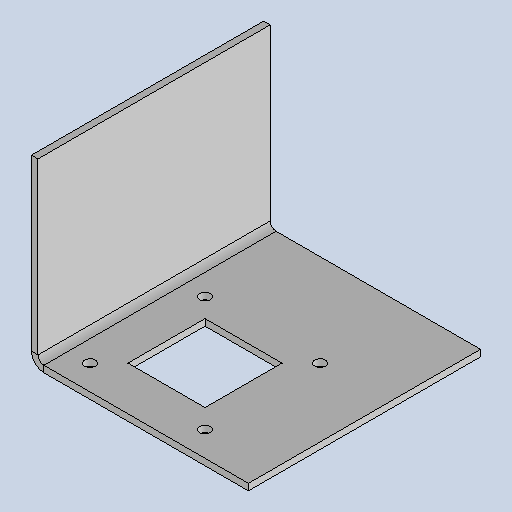
# Autodesk Inventor part: PNS 753 FDS 1200 FLANGE 2 up
Saved by Autodesk Inventor 2025.3 (Build 293356030, 356C)
## iProperties
Created: 2025-06-24
Part Number: PNS 753 FDS 1200 FLANGE 2 up
Material: Stainless Steel
Description: DIE16(5)|\ 90°|corrY -___°|X_____|bom___
Document SubType Name: Sheet Metal
Designer: pokla
Mass: 427.993 g
Surface Area: 379.976 cm^2
Volume: 53.4991 cm^3
Density: 8 g/cm^3
Flat Pattern Width: 17.8893 cm
Flat Pattern Length: 10.7 cm
Flat Pattern Area: 191.416 cm^2
Sheet Metal Rule: AISI304 2mm Die16
Sheet Metal Width: 178,893 mm
Sheet Metal Length: 107,000 mm
Sheet Metal Area: 19141,566 mm^2
Appearance: Default
d177: 30,000 mm
d178: 30,000 mm
Author: user
Autodesk Inventor part; units mm, degrees
ref_plane "YZ Plane" through (0, 0, 0) normal (1, 0, 0) x (0, 1, 0)
ref_plane "XZ Plane" through (0, 0, 0) normal (0, 1, 0) x (-1, 0, 0)
ref_plane "XY Plane" through (0, 0, 0) normal (0, 0, 1) x (1, 0, 0)
sketch "Sketch1" plane through (0, 0, 0) normal (0, 0, 1) x (1, 0, 0)
  line L0 (-50, -53.5) -> (50, -53.5)
  line L1 (50, -53.5) -> (50, 53.5)
  line L2 (50, 53.5) -> (-50, 53.5)
  line L3 (-50, 53.5) -> (-50, -53.5)
  line L4 (-50, -53.5) -> (50, 53.5) construction
  line L5 (50, -53.5) -> (-50, 53.5) construction
  point P0 (0, 0)
  dimension "d154" = 100
  dimension "d155" = 107
  measures "d154" distance of L1.end L2.end
  measures "d155" distance of L0.end L1.end
extrude "Plate5" add sketch "Sketch1" along normal blind 3
sketch "Sketch9" plane through (0, 0, 0) normal (0, 0, -1) x (-1, 0, 0)
  line L0 (25.75, -33.25) -> (-9.75, -33.25)
  line L1 (-9.75, -33.25) -> (-9.75, 2.25)
  line L2 (-9.75, 2.25) -> (25.75, 2.25)
  line L3 (25.75, 2.25) -> (25.75, -33.25)
  line L4 (25.75, -33.25) -> (-9.75, 2.25) construction
  line L5 (-9.75, -33.25) -> (25.75, 2.25) construction
  circle A0 centre (34.5165, -42.0165) radius 2.5
  circle A1 centre (-18.5165, -42.0165) radius 2.5
  circle A2 centre (-18.5165, 11.0165) radius 2.5
  circle A3 centre (34.5165, 11.0165) radius 2.5
  circle A4 centre (8, -15.5) radius 37.5 construction
  line L6 (-9.75, -33.25) -> (-18.5165, -42.0165) construction
  line L7 (50, 53.5) -> (50, -53.5) projected
  line L8 (-50, -53.5) -> (-50, 53.5) projected
  line L9 (50, -53.5) -> (-50, -53.5) projected
  line L10 (50, 53.5) -> (50, -53.5) projected
  line L11 (-50, 53.5) -> (50, 53.5) projected
  point P0 (0, 0)
  dimension "d173" = 35.5
  dimension "d174" = 35.5
  dimension "d175" = 5
  dimension "d176" = 12.3977
  dimension "d179" = 42
  dimension "d180" = 69
  dimension "d183" = 75
  constraints: 14 end point, 5 centre point, 4 point on circle, 4 point on line, 3 equal radius, 2 midpoint, 2 parallel, 1 coincident, 1 horizontal, 1 perpendicular
  measures "d173" distance of L0.start L6.start
  measures "d174" distance of L6.start L1.end
  measures "d175" diameter of A0
  measures "d176" distance of L6.end L6.start
  measures "d179" distance from line of point (8, -15.5) L7
  measures "d180" distance from line of L11 point (8, -15.5)
  measures "d183" diameter of A4
extrude "Extrusion3" cut sketch "Sketch9" against normal blind 10 contours L0 L1 L2 L3 | A0 | A1 | A2 | A3
sketch "Sketch7" plane through (-47, -53.5, 0) normal (-1, 0, 0) x (0, -1, 0)
  line L0 (-107, 0) -> (0, 0)
  line L1 (0, 0) -> (0, 84)
  line L2 (0, 84) -> (-107, 84)
  line L3 (-107, 84) -> (-107, 0)
  constraints: 6 end point, 1 horizontal, 1 perpendicular, 1 vertical
edge flange "Flange3" height 84 angle 90 thickness 3 bend radius 2.75 thickness toward (-1, 0, 0) relief round relief width 3 relief depth 1.5 edges at (-50, 0, 3) wall of the first edge with corners at (-47, 53.5, 0) (-47, -53.5, 0) (-47, -53.5, 84) (-47, 53.5, 84)
bend "Bend3"
corner "Corner3"
body "Solid3"
